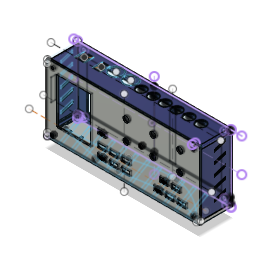
pfm3FrontPanel (Autodesk Fusion 360 design; units mm, degrees)
Autodesk Fusion 360 part; units mm, degrees
sketch "Top face" plane through (0, 0, 0) normal (0, 0, 1) x (1, 0, 0)
  line L0 (0, 0) -> (212.31, 0)
  line L1 (212.31, 0) -> (212.31, 92.645)
  line L2 (212.31, 92.645) -> (0, 92.645)
  line L3 (0, 92.645) -> (0, 0)
  circle A0 centre (9, 6) radius 1.75
  circle A1 centre (203.31, 6) radius 1.75
  line L4 (14.85, 81.85) -> (61.85, 81.85)
  line L5 (61.85, 81.85) -> (61.85, 18.85)
  line L6 (61.85, 18.85) -> (14.85, 18.85)
  line L7 (14.85, 18.85) -> (14.85, 81.85)
  circle A2 centre (110.6, 75.977) radius 4
  circle A3 centre (147.684, 75.977) radius 4
  circle A4 centre (184.768, 75.977) radius 4
  circle A5 centre (110.6, 49.307) radius 4
  circle A6 centre (147.684, 49.307) radius 4
  circle A7 centre (184.768, 49.307) radius 4
  line L8 (82.818, 10.112) -> (70.818, 10.112)
  line L9 (70.818, 10.112) -> (70.818, 16.112)
  line L10 (70.818, 16.112) -> (82.818, 16.112)
  line L11 (82.818, 16.112) -> (82.818, 10.112)
  line L12 (82.818, 10.112) -> (70.818, 16.112) construction
  line L13 (70.818, 10.112) -> (82.818, 16.112) construction
  line L14 (87.328, 16.112) -> (99.328, 16.112)
  line L15 (87.328, 10.112) -> (87.328, 16.112)
  line L16 (99.328, 10.112) -> (87.328, 10.112)
  line L17 (99.328, 16.112) -> (99.328, 10.112)
  line L18 (103.838, 16.112) -> (115.838, 16.112)
  line L19 (103.838, 10.112) -> (103.838, 16.112)
  line L20 (115.838, 10.112) -> (103.838, 10.112)
  line L21 (115.838, 16.112) -> (115.838, 10.112)
  line L22 (70.818, 28.812) -> (82.818, 28.812)
  line L23 (70.818, 22.812) -> (70.818, 28.812)
  line L24 (82.818, 22.812) -> (70.818, 22.812)
  line L25 (82.818, 28.812) -> (82.818, 22.812)
  line L26 (87.328, 28.812) -> (99.328, 28.812)
  line L27 (87.328, 22.812) -> (87.328, 28.812)
  line L28 (99.328, 22.812) -> (87.328, 22.812)
  line L29 (99.328, 28.812) -> (99.328, 22.812)
  line L30 (103.838, 28.812) -> (115.838, 28.812)
  line L31 (103.838, 22.812) -> (103.838, 28.812)
  line L32 (115.838, 22.812) -> (103.838, 22.812)
  line L33 (115.838, 28.812) -> (115.838, 22.812)
  line L34 (82.818, 39.322) -> (70.818, 39.322)
  line L35 (70.818, 39.322) -> (70.818, 45.322)
  line L36 (70.818, 45.322) -> (82.818, 45.322)
  line L37 (82.818, 45.322) -> (82.818, 39.322)
  line L38 (82.818, 39.322) -> (70.818, 45.322) construction
  line L39 (70.818, 39.322) -> (82.818, 45.322) construction
  line L40 (160.288, 10.112) -> (148.288, 10.112)
  line L41 (148.288, 10.112) -> (148.288, 16.112)
  line L42 (148.288, 16.112) -> (160.288, 16.112)
  line L43 (160.288, 16.112) -> (160.288, 10.112)
  line L44 (160.288, 10.112) -> (148.288, 16.112) construction
  line L45 (148.288, 10.112) -> (160.288, 16.112) construction
  line L46 (176.798, 10.112) -> (164.798, 10.112)
  line L47 (176.798, 16.112) -> (176.798, 10.112)
  line L48 (164.798, 10.112) -> (164.798, 16.112)
  line L49 (164.798, 16.112) -> (176.798, 16.112)
  line L50 (193.308, 10.112) -> (181.308, 10.112)
  line L51 (193.308, 16.112) -> (193.308, 10.112)
  line L52 (181.308, 10.112) -> (181.308, 16.112)
  line L53 (181.308, 16.112) -> (193.308, 16.112)
  line L54 (168.543, 24.59) -> (156.543, 24.59)
  line L55 (156.543, 24.59) -> (156.543, 30.59)
  line L56 (156.543, 30.59) -> (168.543, 30.59)
  line L57 (168.543, 30.59) -> (168.543, 24.59)
  line L58 (168.543, 24.59) -> (156.543, 30.59) construction
  line L59 (156.543, 24.59) -> (168.543, 30.59) construction
  line L60 (185.053, 24.59) -> (173.053, 24.59)
  line L61 (173.053, 24.59) -> (173.053, 30.59)
  line L62 (173.053, 30.59) -> (185.053, 30.59)
  line L63 (185.053, 30.59) -> (185.053, 24.59)
  circle A8 centre (131.425, 54.133) radius 2.5
  line L64 (0, -0.028) -> (206.31, -0.028)
  line L65 (-5.2146, 46.3225) -> (227.1425, 46.3225) construction
  line L66 (106.155, 103.4224) -> (106.155, -13.7368) construction
  line L67 (211.08, 1.23) -> (1.23, 1.23)
  line L68 (0, 86.445) -> (0, 91.415)
  circle A9 centre (9, 86.645) radius 1.75
  circle A10 centre (203.31, 86.645) radius 1.75
  line L69 (0, 4.23) -> (3.0548, 4.23)
  line L70 (3.0548, 3.43) -> (1.23, 3.43)
  line L71 (1.23, 3.43) -> (1.23, 1.23)
  line L72 (3.0548, 4.23) -> (3.0548, 3.43)
  line L73 (211.08, 3.43) -> (211.08, 1.23)
  line L74 (209.2552, 3.43) -> (211.08, 3.43)
  line L75 (212.31, 4.23) -> (209.2552, 4.23)
  line L76 (209.2552, 4.23) -> (209.2552, 3.43)
  line L77 (0, 92.645) -> (212.31, 92.645)
  line L78 (212.31, 92.645) -> (212.31, 94.645)
  line L79 (212.31, 94.645) -> (0, 94.645)
  line L80 (0, 94.645) -> (0, 92.645)
  point P0 (9, 6)
  point P1 (66.785, 6)
  point P2 (76.818, 13.112)
  point P3 (76.818, 42.322)
  point P4 (154.288, 13.112)
  point P5 (162.543, 27.59)
  point P6 (131.425, 54.133)
  dimension "d3" = 3.5
  dimension "d4" = 6
  dimension "d5" = 9
  dimension "d11" = 3.5
  dimension "d12" = 194.31
  dimension "d15" = 57.785
  dimension "d16" = 63
  dimension "d17" = 47
  dimension "d20" = 8
  dimension "d23" = 37.084
  dimension "d24" = -26.67
  dimension "d25" = 12
  dimension "d26" = 6
  dimension "d27" = 7.112
  dimension "d28" = 10.033
  dimension "d31" = 16.51
  dimension "d32" = 12.7
  dimension "d34" = 43.815
  dimension "d35" = 69.977
  dimension "d36" = 12
  dimension "d37" = 6
  dimension "d38" = 10.033
  dimension "d39" = 36.322
  dimension "d40" = 12
  dimension "d41" = 6
  dimension "d42" = 7.112
  dimension "d45" = 16.51
  dimension "d46" = 0
  dimension "d47" = 12
  dimension "d48" = 6
  dimension "d51" = 16.51
  dimension "d52" = 0
  dimension "d53" = 21.59
  dimension "d54" = 95.758
  dimension "d60" = 16.51
  dimension "d61" = 16.51
  dimension "d62" = 12.7
  dimension "d63" = 16.51
  dimension "d64" = 16.51
  dimension "d65" = 87.503
  dimension "d69" = 48.133
  dimension "d70" = 64.64
  dimension "d85" = 37.084
  dimension "d86" = 37.084
  dimension "d87" = 26.67
  dimension "d89" = 5
  dimension "d92" = 5.85
  dimension "d93" = 12.85
  dimension "d197" = 9
  dimension "d213" = 1.23
  dimension "d214" = 1.23
  dimension "d216" = 0.8
  dimension "d217" = 2.2
  dimension "d241" = 2
  dimension "d275" = 80.645
  constraint horizontal L0
  constraint vertical L1
  constraint horizontal L2
  constraint vertical L3
  constraint coincident L0.start L3.end
  constraint horizontal P0 P1
  constraint horizontal L4
  constraint vertical L5
  constraint horizontal L6
  constraint vertical L7
  constraint horizontal L8
  constraint perpendicular L8 L9
  constraint parallel L8 L10
  constraint parallel L9 L11
  constraint coincident L12 P2
  constraint coincident L13 P2
  constraint horizontal L34
  constraint perpendicular L34 L35
  constraint parallel L34 L36
  constraint parallel L35 L37
  constraint coincident L38 P3
  constraint coincident L39 P3
  constraint horizontal L40
  constraint perpendicular L40 L41
  constraint parallel L40 L42
  constraint parallel L41 L43
  constraint coincident L44 P4
  constraint coincident L45 P4
  constraint horizontal L54
  constraint perpendicular L54 L55
  constraint parallel L54 L56
  constraint parallel L55 L57
  constraint coincident L58 P5
  constraint coincident L59 P5
  constraint coincident P6 A8.centre
  constraint coincident P0 A0.centre
  constraint horizontal L64
  constraint horizontal L65
  constraint perpendicular L0 L66
  constraint symmetric L0 L2 L65
  constraint symmetric A0 L65 A9
  constraint symmetric A1 L65 A10
  constraint horizontal P0 A1.centre
  constraint perpendicular L3 L69
  constraint perpendicular L3 L70
  constraint perpendicular L67 L71
  constraint perpendicular L70 L72
  constraint symmetric L66 L69.start L75.start
  constraint symmetric L66 L69.end L75.end
  constraint symmetric L66 L70.start L74.start
  constraint symmetric L66 L70.end L73.start
  constraint symmetric L66 L67.end L67.start
  constraint horizontal L77
  constraint vertical L78
  constraint horizontal L79
  constraint vertical L80
  measures "d3" diameter of A0
  measures "d4" distance of L0 P0
  measures "d5" distance of L3 P0
  measures "d11" diameter of A1
  measures "d12" distance of P0 A1.centre
  measures "d15" horizontal distance of P0 P1
  measures "d16" distance of L4.start L6.end
  measures "d17" distance of L4.start L4.end
  measures "d20" diameter of A2
  measures "d25" distance of L9.end L10.end
  measures "d26" distance of L8.end L9.end
  measures "d27" vertical distance of P1 P2
  measures "d28" horizontal distance of P1 P2
  measures "d34" horizontal distance of P1 A2.centre
  measures "d35" vertical distance of P1 A2.centre
  measures "d36" distance of L35.end L36.end
  measures "d37" distance of L34.end L35.end
  measures "d38" horizontal distance of P1 P3
  measures "d39" vertical distance of P1 P3
  measures "d40" distance of L41.end L42.end
  measures "d41" distance of L40.end L41.end
  measures "d42" vertical distance of P1 P4
  measures "d47" distance of L55.end L56.end
  measures "d48" distance of L54.end L55.end
  measures "d53" vertical distance of P1 P5
  measures "d54" horizontal distance of P1 P5
  measures "d60" distance of L23 L27
  measures "d61" distance of L27 L31
  measures "d62" distance of L20 L32
  measures "d63" distance of L41 L48
  measures "d64" distance of L48 L52
  measures "d65" horizontal distance of P1 P4
  measures "d69" vertical distance of P1 P6
  measures "d70" horizontal distance of P1 P6
  measures "d85" distance of A3.centre A4.centre
  measures "d86" distance of A2.centre A3.centre
  measures "d87" distance of A2.centre A5.centre
  measures "d89" diameter of A8
  measures "d92" distance of P0 L7
  measures "d93" distance of P0 L6
  measures "d197" distance of L1 A1.centre
  measures "d213" distance of L0 L67
  measures "d214" distance of L3 L71
  measures "d216" distance of L69 L70
  measures "d217" distance of L67 L70
  measures "d241" distance of L2.end L79.end
  measures "d275" distance of P0 A9.centre
extrude "Extrude1" add sketch "Top face" along normal blind 2 contours L0 L1 L3 L67 L69 L70 L71 L72 L73 L74 L75 L76 | L1 L2 L3 L67 L68 L69 L70 L71 L72 L73 L74 L75 L76 L77 | L2 L77 L78 L79 L80 | A8 makes body 1
extrude "Extrude13" add sketch "Top face" against normal blind 41.3 contours L0 L1 L3 L67 L69 L70 L71 L72 L73 L74 L75 L76 bodies 1
extrude "Extrude5" cut sketch "Top face" along normal blind 1.5 contours A8 bodies 1
sketch "Trou avant" plane through (0, 0, 0) normal (0, -1, 0) x (1, 0, 0)
  line L0 (212.31, -41.3) -> (212.31, 2)
  line L1 (212.31, 2) -> (0, 2)
  line L2 (0, 2) -> (0, -41.3)
  line L3 (0, -41.3) -> (212.31, -41.3)
  line L4 (16.3587, 0.0751) -> (20.3587, 0.0751)
  line L5 (20.3587, 0.0751) -> (6, -39.3751)
  line L6 (6, -39.3751) -> (2, -39.3751)
  line L7 (2, -39.3751) -> (16.3587, 0.0751)
  line L8 (199.3576, -19.65) -> (-44.9421, -19.65) construction
  line L9 (18, -39.3751) -> (32.3587, 0.0751)
  line L10 (32.3587, 0.0751) -> (36.3587, 0.0751)
  line L11 (36.3587, 0.0751) -> (22, -39.3751)
  line L12 (22, -39.3751) -> (18, -39.3751)
  line L13 (34, -39.3751) -> (48.3587, 0.0751)
  line L14 (48.3587, 0.0751) -> (52.3587, 0.0751)
  line L15 (52.3587, 0.0751) -> (38, -39.3751)
  line L16 (38, -39.3751) -> (34, -39.3751)
  line L17 (50, -39.3751) -> (64.3587, 0.0751)
  line L18 (64.3587, 0.0751) -> (68.3587, 0.0751)
  line L19 (68.3587, 0.0751) -> (54, -39.3751)
  line L20 (54, -39.3751) -> (50, -39.3751)
  line L21 (66, -39.3751) -> (80.3587, 0.0751)
  line L22 (80.3587, 0.0751) -> (84.3587, 0.0751)
  line L23 (84.3587, 0.0751) -> (70, -39.3751)
  line L24 (70, -39.3751) -> (66, -39.3751)
  line L25 (82, -39.3751) -> (96.3587, 0.0751)
  line L26 (96.3587, 0.0751) -> (100.3587, 0.0751)
  line L27 (100.3587, 0.0751) -> (86, -39.3751)
  line L28 (86, -39.3751) -> (82, -39.3751)
  line L29 (98, -39.3751) -> (112.3587, 0.0751)
  line L30 (112.3587, 0.0751) -> (116.3587, 0.0751)
  line L31 (116.3587, 0.0751) -> (102, -39.3751)
  line L32 (102, -39.3751) -> (98, -39.3751)
  line L33 (114, -39.3751) -> (128.3587, 0.0751)
  line L34 (128.3587, 0.0751) -> (132.3587, 0.0751)
  line L35 (132.3587, 0.0751) -> (118, -39.3751)
  line L36 (118, -39.3751) -> (114, -39.3751)
  line L37 (130, -39.3751) -> (144.3587, 0.0751)
  line L38 (144.3587, 0.0751) -> (148.3587, 0.0751)
  line L39 (148.3587, 0.0751) -> (134, -39.3751)
  line L40 (134, -39.3751) -> (130, -39.3751)
  line L41 (146, -39.3751) -> (160.3587, 0.0751)
  line L42 (160.3587, 0.0751) -> (164.3587, 0.0751)
  line L43 (164.3587, 0.0751) -> (150, -39.3751)
  line L44 (150, -39.3751) -> (146, -39.3751)
  spline S0 degree 5 poles (4.3333, -21.1869) (7.9803, -19.9926) (15.1629, -17.7257) (25.6024, -14.6899) (38.8481, -11.3765) (54.2633, -8.477) (68.5311, -6.8192) (81.683, -6.3544) (93.8129, -6.9567) (105.113, -8.3801) (115.8931, -10.2369) (126.5121, -12.0803) (137.3257, -13.4705) (148.63, -14.0437) (160.6015, -13.5881) (173.3264, -12.0047) (184.132, -9.8135) (192.5869, -7.6538) (198.3783, -5.9863) (201.3127, -5.0956) knots 0 0 0 0 0 0 0.066667 0.133333 0.2 0.266667 0.333333 0.4 0.466667 0.533333 0.6 0.666667 0.733333 0.8 0.866667 0.933333 1 1 1 1 1 1
  spline S1 degree 5 poles (201.3127, -5.0956) (198.9381, -7.4107) (194.1855, -11.8338) (187.0464, -17.8473) (177.5072, -24.614) (165.5442, -30.9528) (153.5289, -35.1651) (141.4358, -37.3159) (129.2234, -37.5939) (116.8297, -36.3675) (104.1823, -34.1052) (91.2085, -31.3047) (77.8443, -28.4285) (64.0482, -25.8275) (49.8059, -23.7077) (35.1179, -22.1797) (23.0176, -21.4642) (13.7498, -21.2147) (7.4863, -21.175) (4.3333, -21.1869) knots 0 0 0 0 0 0 0.066667 0.133333 0.2 0.266667 0.333333 0.4 0.466667 0.533333 0.6 0.666667 0.733333 0.8 0.866667 0.933333 1 1 1 1 1 1
  line L45 (162, -39.3751) -> (176.3587, 0.0751)
  line L46 (176.3587, 0.0751) -> (180.3587, 0.0751)
  line L47 (180.3587, 0.0751) -> (166, -39.3751)
  line L48 (166, -39.3751) -> (162, -39.3751)
  line L49 (178, -39.3751) -> (192.3587, 0.0751)
  line L50 (192.3587, 0.0751) -> (196.3587, 0.0751)
  line L51 (196.3587, 0.0751) -> (182, -39.3751)
  line L52 (182, -39.3751) -> (178, -39.3751)
  point P0 (138.1297, -13.3249)
  point P1 (141.8381, -36.804)
  point P2 (82.6115, -29.4903)
  point P3 (91.1793, -6.9755)
  dimension "d257" = 4
  dimension "d259" = 70
  dimension "d262" = 16
  dimension "d263" = 0
  dimension "d264" = 2
  constraint horizontal L4
  constraint horizontal L6
  constraint parallel L5 L7
  constraint perpendicular L2 L8
  measures "d257" distance of L4.start L4.end
  measures "d259" angle of L6 L7
  measures "d264" distance of L2 L6.end
fillet "Fillet3" radius 2 1 edges at (106.155, 1.23, 0) on bodies 1
fillet "Fillet4" radius 2 2 edges at (0, 94.645, 1) (212.31, 94.645, 1) on bodies 1
ref_plane "WorkPlane2" through (106.155, 47.3225, -41.6) normal (0, 0, -1) x (-1, 0, 0)
sketch "Bottom" plane through (103.155, 46.3225, -41.6) normal (0, 0, -1) x (1, 0, 0)
  line L0 (109.155, 46.3225) -> (109.155, -46.3225)
  line L1 (-103.155, 46.3505) -> (103.155, 46.3505)
  circle A0 centre (100.155, 40.3225) radius 1.75
  circle A1 centre (-94.155, 40.3225) radius 1.75
  line L2 (-103.155, -46.3225) -> (-103.155, 46.3225)
  line L3 (109.155, -46.3225) -> (-103.155, -46.3225)
  line L4 (-108.3696, 0) -> (123.9875, 0) construction
  line L5 (3, -57.0999) -> (3, 60.0593) construction
  line L6 (-101.925, 40.4625) -> (-101.925, -45.0925)
  line L7 (-103.155, -46.3225) -> (-103.155, 41.6925)
  line L8 (3, -45.0925) -> (-101.925, -45.0925)
  line L9 (3, -45.0925) -> (107.925, -45.0925)
  circle A2 centre (100.155, -40.3225) radius 1.75
  circle A3 centre (-94.155, -40.3225) radius 1.75
  line L10 (-103.155, 46.3225) -> (109.155, 46.3225)
  line L11 (-101.925, 34.5925) -> (-99.925, 34.5925)
  line L12 (-99.925, 34.5925) -> (-99.925, 35.8225)
  line L13 (-99.925, 35.8225) -> (-101.925, 35.8225)
  line L14 (-101.925, 35.8225) -> (-101.925, 34.5925)
  line L15 (107.925, 34.5925) -> (105.925, 34.5925)
  line L16 (105.925, 34.5925) -> (105.925, 35.8225)
  line L17 (105.925, 35.8225) -> (107.925, 35.8225)
  line L18 (-89.925, -33.0925) -> (3, -33.0925)
  line L19 (3, -33.0925) -> (3, 33.0925)
  line L20 (3, 33.0925) -> (-89.925, 33.0925)
  line L21 (-89.925, 33.0925) -> (-89.925, -33.0925)
  line L22 (95.925, -33.0925) -> (3, -33.0925)
  line L23 (95.925, 33.0925) -> (95.925, -33.0925)
  line L24 (3, 33.0925) -> (95.925, 33.0925)
  line L25 (-101.925, 34.5925) -> (107.925, 34.5925)
  line L26 (107.925, 34.5925) -> (107.925, 35.8225)
  line L27 (107.925, 35.8225) -> (-101.925, 35.8225)
  line L28 (-101.925, 35.8225) -> (-101.925, 34.5925)
  line L29 (-101.925, 40.4625) -> (-97.7681, 40.4625)
  line L30 (-97.7681, 40.4625) -> (-97.7681, 44.5225)
  line L31 (-97.7681, 44.5225) -> (-101.155, 44.5225)
  line L32 (-101.155, 44.5225) -> (-101.155, 43.2925)
  line L33 (-101.155, 43.2925) -> (-98.9981, 43.2925)
  line L34 (-98.9981, 43.2925) -> (-98.9981, 41.6925)
  line L35 (-98.9981, 41.6925) -> (-103.155, 41.6925)
  line L36 (-103.155, 42.0925) -> (-100.1002, 42.0925)
  line L37 (107.925, 40.4625) -> (107.925, -45.0925)
  line L38 (107.925, 40.4625) -> (103.7681, 40.4625)
  line L39 (103.7681, 40.4625) -> (103.7681, 44.5225)
  line L40 (103.7681, 44.5225) -> (107.155, 44.5225)
  line L41 (107.155, 44.5225) -> (107.155, 43.2925)
  line L42 (107.155, 43.2925) -> (106.8604, 43.0322)
  line L43 (107.155, 43.2925) -> (104.9981, 43.2925)
  line L44 (104.9981, 43.2925) -> (104.9981, 41.6925)
  line L45 (104.9981, 41.6925) -> (109.155, 41.6925)
  line L46 (106.8604, 43.0322) -> (107.155, 43.2925)
  line L47 (-101.925, 40.4625) -> (-101.925, 41.6925)
  line L48 (107.925, 40.4625) -> (107.925, 41.6925)
  line L49 (-100.1002, 42.8925) -> (-101.925, 42.8925)
  line L50 (28.405, -54.8343) -> (28.405, 50.5338) construction
  line L51 (24.405, -33.0925) -> (32.405, -33.0925)
  line L52 (32.405, -33.0925) -> (32.405, 33.0925)
  line L53 (32.405, 33.0925) -> (24.405, 33.0925)
  line L54 (24.405, 33.0925) -> (24.405, -33.0925)
  dimension "d187" = 1.23
  dimension "d199" = 2
  dimension "d200" = 1.23
  dimension "d202" = 104.955
  dimension "d205" = 12
  dimension "d206" = 12
  dimension "d207" = 1.23
  dimension "d209" = 4.5
  dimension "d212" = 1.23
  dimension "d220" = 90
  dimension "d221" = 0.4
  dimension "d222" = 1.23
  dimension "d223" = 1.23
  dimension "d224" = 1.23
  dimension "d237" = 2
  dimension "d238" = 0.4
  dimension "d255" = 71.75
  dimension "d256" = 8
  constraint vertical L6
  constraint vertical L7
  constraint coincident L2 L7.end
  constraint horizontal L8
  constraint coincident L5 L8.start
  constraint symmetric L5 L8.start L9.start
  constraint symmetric L5 L6.end L9.end
  constraint horizontal L11
  constraint vertical L12
  constraint horizontal L13
  constraint vertical L14
  constraint symmetric L5 L11.start L15.start
  constraint symmetric L5 L11.end L15.end
  constraint symmetric L5 L12.end L16.end
  constraint symmetric L5 L13.end L17.end
  constraint horizontal L18
  constraint vertical L19
  constraint horizontal L20
  constraint vertical L21
  constraint coincident L5 L19.end
  constraint symmetric L4 L18 L20
  constraint symmetric L5 L18.start L22.start
  constraint symmetric L5 L18.end L19.start
  constraint symmetric L5 L19.end L20.start
  constraint symmetric L5 L20.end L23.start
  constraint horizontal L25
  constraint vertical L26
  constraint horizontal L27
  constraint vertical L28
  constraint coincident L6 L11.start
  constraint perpendicular L6 L29
  constraint perpendicular L29 L30
  constraint perpendicular L30 L31
  constraint perpendicular L31 L32
  constraint coincident L7 L35.end
  constraint symmetric L5 L6.start L37.start
  constraint symmetric L5 L29.end L38.end
  constraint symmetric L5 L30.end L39.end
  constraint symmetric L5 L31.end L40.end
  constraint symmetric L5 L32.end L41.end
  constraint symmetric L5 L33.end L43.end
  constraint symmetric L5 L34.end L44.end
  constraint symmetric L5 L7.end L45.end
  constraint coincident L35 L47.end
  constraint perpendicular L35 L47
  constraint coincident L45 L48.end
  constraint perpendicular L45 L48
  constraint coincident L13.end L14.start
  constraint vertical L50
  constraint horizontal L51
  constraint vertical L52
  constraint horizontal L53
  constraint vertical L54
  constraint coincident L24 L52.end
  constraint coincident L22 L51.start
  constraint symmetric L50 L52 L54
  measures "d187" distance of L6 L7
  measures "d199" distance of L11.start L11.end
  measures "d200" distance of L11.start L13.end
  measures "d205" distance of L9 L22
  measures "d206" distance of L6 L21
  measures "d207" distance of L25 L27
  measures "d209" distance of A0.centre L27
  measures "d212" distance of L3 L8
  measures "d220" angle of L34 L35
  measures "d221" distance of L35 L36
  measures "d222" distance of L29 L35
  measures "d223" distance of L30 L34
  measures "d224" distance of L31 L33
  measures "d237" distance of L2 L32
  measures "d238" distance of L33 L49
  measures "d255" distance of A2.centre L50
  measures "d256" distance of L52 L54
extrude "Extrude17" add sketch "Bottom" along normal blind 2 separate body contours L0 L2 L6 L10 L13 L17 L27 L29 L30 L31 L32 L33 L34 L35 L37 L38 L39 L40 L41 L43 L44 L45 | L0 L2 L3 L6 L7 L8 L9 L14 L26 L28 L35 L37 L45 L47 L48 | L38 L39 L40 L41 L43 L44 L45 L48 | L15 L16 L17 L25 L26 L27 L37 | L29 L30 L31 L32 L33 L34 L35 L47 | L12 L16 L25 L27 | L6 L8 L9 L11 L15 L25 L37 | L6 L11 L12 L13 L14 L25 L27 L28 | L22 L24 L51 L52 L53 L54 makes body 2
extrude "Extrude18" add sketch "Bottom" against normal blind 41.5 contours L0 L2 L3 L6 L7 L8 L9 L14 L26 L28 L35 L37 L45 L47 L48 | L15 L16 L17 L25 L26 L27 L37 | L6 L11 L12 L13 L14 L25 L27 L28 bodies 2
extrude "Extrude20" add sketch "Bottom" against normal blind 2 contours L15 L16 L17 L25 L26 L27 L37 | L12 L16 L25 L27 | L6 L11 L12 L13 L14 L25 L27 L28 bodies 2
extrude "Extrude21" add sketch "Bottom" against normal blind 6 contours L38 L39 L40 L41 L43 L44 L45 L48 | L29 L30 L31 L32 L33 L34 L35 L47 bodies 2
sketch "Back face" plane through (0, 92.645, 0) normal (0, 1, 0) x (-1, 0, 0)
  line L0 (16.6542, -21.6) -> (-218.1831, -21.6) construction
  circle A0 centre (-184.269, -28.1) radius 6.5
  circle A1 centre (-167.759, -28.1) radius 6.5
  circle A2 centre (-151.249, -28.1) radius 6.5
  circle A3 centre (-134.739, -28.1) radius 6.5
  circle A4 centre (-118.229, -28.1) radius 6.5
  circle A5 centre (-101.719, -28.1) radius 6.5
  circle A6 centre (-83.764, -31.61) radius 9
  circle A7 centre (-63.444, -31.61) radius 9
  line L1 (-42.569, -20.6) -> (-52.569, -20.6)
  line L2 (-52.569, -20.6) -> (-52.569, -33.6)
  line L3 (-52.569, -33.6) -> (-42.569, -33.6)
  line L4 (-42.569, -33.6) -> (-42.569, -20.6)
  line L5 (-42.569, -20.6) -> (-52.569, -33.6) construction
  line L6 (-52.569, -20.6) -> (-42.569, -33.6) construction
  line L7 (-17.554, -33.2) -> (-30.594, -33.2)
  line L8 (-30.594, -33.2) -> (-30.594, -20.6)
  line L9 (-30.594, -20.6) -> (-17.554, -20.6)
  line L10 (-17.554, -20.6) -> (-17.554, -33.2)
  line L11 (-17.554, -33.2) -> (-30.594, -20.6) construction
  line L12 (-30.594, -33.2) -> (-17.554, -20.6) construction
  line L13 (5.2146, -41.6) -> (-227.1425, -41.6)
  line L14 (-203.31, -1) -> (-203.31, 3)
  point P0 (-47.569, -27.1)
  point P1 (-24.074, -26.9)
  dimension "d110" = 13
  dimension "d111" = 6.5
  dimension "d115" = 16.51
  dimension "d116" = 0
  dimension "d118" = 18
  dimension "d119" = 10.01
  dimension "d122" = 20.32
  dimension "d123" = 0
  dimension "d124" = 16.51
  dimension "d125" = 20.32
  dimension "d126" = 10
  dimension "d127" = 13
  dimension "d129" = 1
  dimension "d130" = 13.04
  dimension "d131" = 12.6
  dimension "d133" = 1
  dimension "d193" = 20
  dimension "d239" = 19.041
  constraint horizontal L1
  constraint perpendicular L1 L2
  constraint parallel L1 L3
  constraint parallel L2 L4
  constraint coincident L5 P0
  constraint coincident L6 P0
  constraint horizontal L7
  constraint perpendicular L7 L8
  constraint parallel L7 L9
  constraint parallel L8 L10
  constraint coincident L11 P1
  constraint coincident L12 P1
  measures "d110" diameter of A0
  measures "d111" distance of L0 A0.centre
  measures "d118" diameter of A6
  measures "d119" distance of L0 A6.centre
  measures "d124" distance of A0.centre A1.centre
  measures "d125" distance of A6.centre A7.centre
  measures "d126" distance of L2.end L3.end
  measures "d127" distance of L1.end L2.end
  measures "d129" distance of L0 L1
  measures "d130" distance of L8.end L9.end
  measures "d131" distance of L7.end L8.end
  measures "d133" distance of L0 L9
  measures "d193" distance of L0 L13
  measures "d239" distance of A0.centre L14
extrude "Extrude19" cut sketch "Back face" against normal up to surface (1.23 mm away) bodies 2
sketch "SD" plane through (0, 0, 0) normal (-1, 0, 0) x (0, 0, 1)
  line L0 (-0.1, 92.645) -> (-43.6, 92.645)
  line L1 (-43.6, 92.645) -> (-43.6, 0)
  line L2 (-43.6, 0) -> (-41.6, 0)
  line L3 (-41.6, 0) -> (-41.6, 4.63)
  line L4 (-41.6, 4.63) -> (-0.1, 4.63)
  line L5 (-0.1, 4.63) -> (-0.1, 92.645)
  line L6 (-5.1, 67.645) -> (-11.1, 67.645)
  line L7 (-11.1, 67.645) -> (-11.1, 37.645)
  line L8 (-11.1, 37.645) -> (-5.1, 37.645)
  line L9 (-5.1, 37.645) -> (-5.1, 67.645)
  line L10 (-34.1863, 85.46) -> (-18.7339, 80.6115)
  line L11 (-18.7339, 80.6115) -> (-18.7339, 77.6115)
  line L12 (-18.7339, 77.6115) -> (-34.1863, 82.46)
  line L13 (-34.1863, 82.46) -> (-34.1863, 85.46)
  line L14 (-34.1863, 67.46) -> (-34.1863, 70.46)
  line L15 (-34.1863, 70.46) -> (-18.7339, 65.6115)
  line L16 (-18.7339, 65.6115) -> (-18.7339, 62.6115)
  line L17 (-18.7339, 62.6115) -> (-34.1863, 67.46)
  line L18 (-34.1863, 52.46) -> (-34.1863, 55.46)
  line L19 (-34.1863, 55.46) -> (-18.7339, 50.6115)
  line L20 (-18.7339, 50.6115) -> (-18.7339, 47.6115)
  line L21 (-18.7339, 47.6115) -> (-34.1863, 52.46)
  line L22 (-34.1863, 37.46) -> (-34.1863, 40.46)
  line L23 (-34.1863, 40.46) -> (-18.7339, 35.6115)
  line L24 (-18.7339, 35.6115) -> (-18.7339, 32.6115)
  line L25 (-18.7339, 32.6115) -> (-34.1863, 37.46)
  line L26 (-34.1863, 22.46) -> (-34.1863, 25.46)
  line L27 (-34.1863, 25.46) -> (-18.7339, 20.6115)
  line L28 (-18.7339, 20.6115) -> (-18.7339, 17.6115)
  line L29 (-18.7339, 17.6115) -> (-34.1863, 22.46)
  dimension "d232" = 5
  dimension "d233" = 6
  dimension "d234" = 25
  dimension "d235" = 30
  dimension "d267" = 3
  dimension "d270" = 0
  dimension "d271" = -15
  constraint horizontal L6
  constraint vertical L7
  constraint horizontal L8
  constraint vertical L9
  constraint vertical L11
  constraint vertical L13
  constraint parallel L10 L12
  measures "d232" distance of L5 L9
  measures "d233" distance of L7 L9
  measures "d234" distance of L0 L6
  measures "d235" distance of L6 L8
  measures "d267" distance of L10.end L11.end
extrude "Extrude25" cut sketch "SD" against normal up to surface (212.31 mm away) contours L10 L11 L12 L13 | L14 L15 L16 L17 | L18 L19 L20 L21 | L22 L23 L24 L25 | L26 L27 L28 L29 bodies 2
extrude "Extrude22" cut sketch "SD" against normal up to surface (1.23 mm away) contours L6 L7 L8 L9 bodies 2
extrude "Extrude24" cut sketch "Trou avant" against normal up to surface (1.23 mm away) contours L5 L7 S0 S1 | L9 L11 S0 S1 | L13 L15 S0 S1 | L17 L19 S0 S1 | L21 L23 S0 S1 | L25 L27 S0 S1 | L29 L31 S0 S1 | L33 L35 S0 S1 | L37 L39 S0 S1 | L41 L43 S0 S1 | S0 S1 L45 L47 | S0 S1 L49 L51 bodies 1
fillet "Fillet5" radius 3 4 edges at (1.23, 91.415, -20.85) (0, 92.645, -21.85) (212.31, 92.645, -21.85) (211.08, 91.415, -20.85) on bodies 2
equation "d239 = 23.241 mm - 4.2 mm"
named bodies: "Top", "Bottom"
